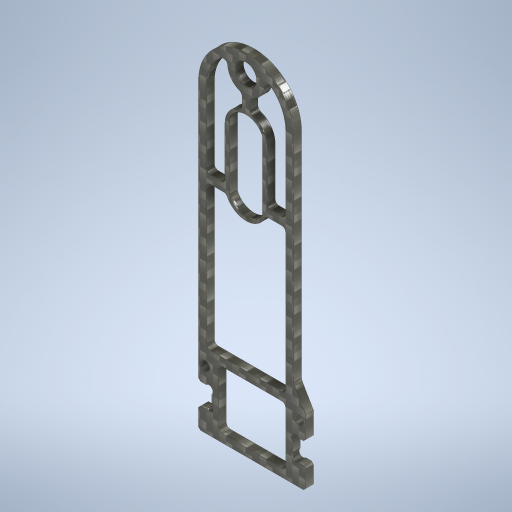
# Autodesk Inventor part: UpperArmFrame
Saved by Autodesk Inventor 2024.2 (Build 282272000, 272)
## iProperties
Created: 2024-01-18
Part Number: UpperArmFrame
Material: CFRP
Document SubType Name: Modeling
Designer: Masato Kubotera
Density: 1.43 g/cm^3
Appearance: Carbon Fiber 1
Mass: 8.48663 g
Surface Area: 72.2235 cm^2
Volume: 5.9347 cm^3
Vendor: ALLPCB
Author: Masato Kubotera
Autodesk Inventor part; units mm, degrees
ref_plane "YZ Plane" through (0, 0, 0) normal (1, 0, 0) x (0, 1, 0)
ref_plane "XZ Plane" through (0, 0, 0) normal (0, 1, 0) x (-1, 0, 0)
ref_plane "XY Plane" through (0, 0, 0) normal (0, 0, 1) x (1, 0, 0)
sketch "Sketch1" plane through (0, 0, 0) normal (1, 0, 0) x (0, 1, 0)
  arc A0 (6.25, -17.1964) -> (-6.25, -17.1964) centre (0, -20) ccw
  line L0 (-6.25, -17.1964) -> (-6.25, -42.8036)
  line L1 (-6.25, -30) -> (6.25, -30) construction
  line L2 (0, 0) -> (0, -137.3205) construction
  arc A1 (-6.25, -42.8036) -> (6.25, -42.8036) centre (0, -40) ccw
  circle A2 centre (0, 0) radius 40 construction
  circle A3 centre (0, -20) radius 20 construction
  line L3 (6.25, -17.1964) -> (6.25, -42.8036)
  line L4 (0, 0) -> (17.3205, -10) construction
  line L5 (17.3205, -10) -> (34.641, -20) construction
  line L6 (-25, -137.3205) -> (25, -137.3205) construction
  line L7 (-18, -125.3205) -> (-18, -29)
  line L8 (22.5, -125.3205) -> (22.5, -100.3205)
  line L9 (-25, -120) -> (25, -120) construction
  line L10 (25, -120) -> (25, -137.3205) construction
  line L11 (-25, -120) -> (-25, -137.3205) construction
  line L12 (22.5, -109.2705) -> (17.5, -109.2705)
  line L13 (17.5, -109.2705) -> (17.5, -117.3705)
  line L14 (17.5, -117.3705) -> (22.5, -117.3705)
  line L15 (-15, -106.3205) -> (17.5, -106.3205) construction
  line L16 (17.5, -106.3205) -> (17.5, -149.3205) construction
  line L17 (17.5, -149.3205) -> (-15, -149.3205) construction
  line L18 (-15, -149.3205) -> (-15, -106.3205) construction
  line L19 (-15, -106.3205) -> (17.5, -149.3205) construction
  line L20 (17.5, -106.3205) -> (-15, -149.3205) construction
  line L21 (1.25, -106.3205) -> (1.25, -149.3205) construction
  line L22 (22.5, -109.3205) -> (17.5, -109.3205) construction
  line L23 (17.5, -117.3205) -> (22.5, -117.3205) construction
  line L24 (17.5, -113.3205) -> (22.5, -113.3205) construction
  line L25 (-18, -100.3205) -> (22.5, -100.3205) construction
  circle A4 centre (0, 0) radius 4 construction
  circle A5 centre (20, -103.3205) radius 1.75 construction
  line L26 (20, -103.3205) -> (20, -123.3205) construction
  circle A6 centre (20, -123.3205) radius 1.75 construction
  line L27 (-18, -109.2705) -> (-13, -109.2705)
  line L28 (-13, -109.2705) -> (-13, -117.3705)
  line L29 (-13, -117.3705) -> (-18, -117.3705)
  line L30 (-15.5, -103.3205) -> (-15.5, -123.3205) construction
  line L31 (-15.5, -103.3205) -> (20, -103.3205) construction
  line L32 (-15.5, -123.3205) -> (20, -123.3205) construction
  arc A7 (-4.4, -42.3749) -> (4.4, -42.3749) centre (0, -40) ccw construction
  arc A8 (4.4, -17.6251) -> (-4.4, -17.6251) centre (0, -20) ccw construction
  line L33 (-4.4, -17.6251) -> (-4.4, -42.3749) construction
  line L34 (4.4, -42.3749) -> (4.4, -17.6251) construction
  line L35 (-18, -29) -> (-18, -11)
  circle A9 centre (0, 0) radius 7 construction
  arc A10 (18, -11) -> (-18, -11) centre (0, -11) ccw
  line L36 (18, -11) -> (18, -92.5263)
  line L37 (18, -92.5263) -> (22.5, -100.3205)
  line L38 (-15, -42.8036) -> (-15, -97.3205)
  line L39 (-15, -97.3205) -> (15, -97.3205)
  line L40 (15, -42.8036) -> (15, -97.3205)
  line L41 (-10.5, -100.3205) -> (15, -100.3205)
  line L42 (15, -100.3205) -> (15, -122.3205)
  line L43 (15, -122.3205) -> (-10.5, -122.3205)
  line L44 (-10.5, -122.3205) -> (-10.5, -100.3205)
  line L45 (-15, -39.8036) -> (-8, -39.8036)
  arc A11 (-6.5383, 2.5) -> (-15, -11) centre (0, -11) ccw
  arc A12 (-6.5383, 2.5) -> (-1.5, -6.8374) centre (0, 0) ccw
  line L46 (-15, -11) -> (-15, -39.8036)
  line L47 (8, -39.8036) -> (8, -20)
  line L48 (15, -39.8036) -> (8, -39.8036)
  arc A13 (15, -11) -> (6.5383, 2.5) centre (0, -11) ccw
  arc A14 (1.5, -6.8374) -> (6.5383, 2.5) centre (0, 0) ccw
  line L49 (15, -11) -> (15, -39.8036)
  arc A15 (-7.4927, -42.8036) -> (7.4927, -42.8036) centre (0, -40) ccw
  line L50 (-15, -42.8036) -> (-7.4927, -42.8036)
  line L51 (-8, -39.8036) -> (-8, -20)
  arc A16 (-1.5, -12.1419) -> (-8, -20) centre (0, -20) ccw
  line L52 (-1.5, -6.8374) -> (-1.5, -12.1419)
  line L53 (15, -42.8036) -> (7.4927, -42.8036)
  arc A17 (8, -20) -> (1.5, -12.1419) centre (0, -20) ccw
  line L54 (1.5, -6.8374) -> (1.5, -12.1419)
  line L55 (-18, -137.3205) -> (-18, -100.3205) construction
  circle A18 centre (-15.5, -103.3205) radius 1.75 construction
  line L56 (22.5, -100.3205) -> (22.5, -137.3205) construction
  line L57 (-18, -125.3205) -> (22.5, -125.3205)
  arc A19 (19.6213, -109.2705) -> (17.5, -111.3918) centre (18.5607, -110.3312) ccw
  arc A20 (17.5, -115.2492) -> (19.6213, -117.3705) centre (18.5607, -116.3098) ccw
  arc A21 (-13, -111.3918) -> (-15.1213, -109.2705) centre (-14.0607, -110.3312) ccw
  arc A22 (-15.1213, -117.3705) -> (-13, -115.2492) centre (-14.0607, -116.3098) ccw
  line L58 (2.25, -122.3205) -> (2.25, -100.3205) construction
  point P0 (5.3819, -44.2376)
  point P1 (6.25, -41.5156)
  point P2 (17.5, -112.2705)
  point P3 (17.5, -114.3705)
  point P4 (1.25, -127.8205)
  point P5 (-13, -111.3918)
  point P6 (-13, -114.8191)
  point P7 (8, -20)
  point P8 (-13, -115.2492)
  point P9 (19.6213, -117.3705)
  point P10 (17.5, -115.2492)
  point P11 (17.5, -111.3918)
  dimension "d2" = 12.5
  dimension "d3" = 60
  dimension "d4" = 20
  dimension "d5" = 20
  dimension "d6" = 20
  dimension "d12" = 17.3205
  dimension "d13" = 120
  dimension "d17" = 32.5
  dimension "d18" = 43
  dimension "d19" = 9.5
  dimension "d21" = 0.05
  dimension "d24" = 3
  dimension "d25" = 9
  dimension "d26" = 6
  dimension "d36" = 8
  dimension "d48" = 50
  dimension "d50" = 3
  dimension "d51" = 3.5
  dimension "d56" = 8.8
  dimension "d57" = 5
  dimension "d58" = 1.85
  dimension "d59" = 1.85
  dimension "d65" = 14
  dimension "d66" = 30
  dimension "d70" = 3
  dimension "d74" = 3
  dimension "d78" = 1.75
  dimension "d81" = 7
  dimension "d82" = 5
  dimension "d85" = 5
  dimension "d86" = 2.5
  dimension "d91" = 8
  dimension "d92" = 8
  dimension "d93" = 3
  dimension "d95" = 3
  dimension "d96" = 3
  dimension "d97" = 8
  dimension "d99" = 1.5
  constraints: 120 end point, 41 point on circle, 28 point on line, 23 centre point, 23 symmetric about line, 18 horizontal, 18 vertical, 12 coincident, 10 midpoint, 7 collinear, 5 equal radius, 4 parallel, 4 tangent, 2 concentric, 2 perpendicular, 13 other
  measures "d2" distance between parallel lines of L3 L0
  measures "d3" angle of L4 L2
  measures "d4" distance of L4.end L5.end
  measures "d5" radius of A3
  measures "d6" distance of A1.centre A0.centre
  measures "d12" distance between parallel lines of L6 L9
  measures "d13" distance from line of L9 A3.end
  measures "d17" distance of L16.end L17.end
  measures "d18" distance of L15.end L16.end
  measures "d19" distance from line of L6 point (1.25, -127.821)
  measures "d21" distance between parallel lines of L22 L12
  measures "d24" distance between parallel lines of L22 L15
  measures "d25" distance between parallel lines of L22 L25
  measures "d26" distance from line of point (20, -103.321) L22
  measures "d36" diameter of A4
  measures "d48" distance between parallel lines of L10 L11
  measures "d50" distance between parallel lines of L18 L7
  measures "d51" diameter of A5
  measures "d56" distance between parallel lines of L34 L33
  measures "d57" radius of A8
  measures "d58" distance between parallel lines of L3 L34
  measures "d59" radial gap between concentric circles of A1 A7
  measures "d65" diameter of A9
  measures "d66" angle of L36 L37
  measures "d70" radial gap between concentric circles of A10 A11
  measures "d74" distance between parallel lines of L41 L39
  measures "d78" distance between parallel lines of L0 L51
  measures "d81" distance between parallel lines of L11 L55
  measures "d82" distance between parallel lines of L28 L55
  measures "d85" distance between parallel lines of L13 L56
  measures "d86" distance between parallel lines of L10 L56
  measures "d91" distance between parallel lines of L23 L22
  measures "d92" distance between parallel lines of L57 L23
  measures "d93" distance between parallel lines of L57 L43
  measures "d95" distance between parallel lines of L50 L45
  measures "d96" distance between parallel lines of L54 L52
  measures "d97" radius of A15
  measures "d99" radius of A19
extrude "Extrusion1" add sketch "Sketch1" along normal blind 3 contours L7 L29 A22 L28 A21 L27 L35 A10 L36 L37 L8 L12 A19 L13 A20 L14 L57
hole "Hole1" at (0, 0, 0) direction (1, 0, 0) diameter 8 end through all
hole "Hole2" at (0, 20, -103.3205) at (0, -15.5, -103.3205) direction (1, 0, 0) diameter 3.5 end through all
fillet "Fillet1" radius 2 5 edges at (1.5, -6.25, -17.1964) (1.5, -6.25, -42.8036) (1.5, 6.25, -42.8036) (1.5, 6.25, -17.1964) (1.5, 18, -92.5263)
fillet "Fillet2" radius 1.5 20 edges at (1.5, -6.5383, 2.5) (1.5, -1.5, -6.8374) (1.5, 6.5383, 2.5) (1.5, -8, -39.8036) (1.5, -15, -39.8036) (1.5, -15, -42.8036) (1.5, 15, -39.8036) (1.5, 8, -39.8036) (1.5, 15, -42.8036) (1.5, 15, -100.3205) (1.5, 15, -97.3205) (1.5, -15, -97.3205) (1.5, -10.5, -100.3205) (1.5, -10.5, -122.3205) (1.5, 15, -122.3205) (1.5, -7.4927, -42.8036) (1.5, 7.4927, -42.8036) (1.5, 1.5, -12.1419) (1.5, -1.5, -12.1419) (1.5, 1.5, -6.8374)
chamfer "Chamfer1" distance 0.75 angle 45 6 edges at (1.5, 22.5, -109.2705) (1.5, 22.5, -117.3705) (1.5, -18, -117.3705) (1.5, -18, -109.2705) (1.5, -18, -125.3205) (1.5, 22.5, -125.3205)
equation "\"d6\" = d4"
body "Solid1"
